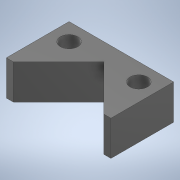
# Autodesk Inventor part: Subj_Cube
Saved by Autodesk Inventor 2021 (Build 250183000, 183)
## iProperties
Created: 2021-05-07
Part Number: Subj_Cube
Material: Genérico
Document SubType Name: Modeling
Designer: Marc
Density: 1 g/cm^3
Appearance: Valor por defecto
Author: Marc
## iProperties of the stored document _3DPrint.ipt
Created: 2021-05-07
Part Number: _3DPrint
Material: Genérico
Document SubType Name: Modeling
Designer: Marc
Density: 1 g/cm^3
Appearance: Valor por defecto
Author: Marc
Autodesk Inventor part; units mm, degrees
ref_plane "YZ Plane" through (0, 0, 0) normal (1, 0, 0) x (0, 1, 0)
ref_plane "XZ Plane" through (0, 0, 0) normal (0, 1, 0) x (-1, 0, 0)
ref_plane "XY Plane" through (0, 0, 0) normal (0, 0, 1) x (1, 0, 0)
sketch "Boceto1" plane through (0, 0, 0) normal (0, 1, 0) x (-1, 0, 0)
  line L0 (-15, -10) -> (15, -10)
  line L1 (13, 8) -> (0, -5)
  line L2 (-13, 8) -> (0, -5)
  line L3 (-15, 8) -> (-13, 8)
  line L4 (15, 8) -> (13, 8)
  line L5 (15, -10) -> (15, 8)
  line L6 (-15, -10) -> (-15, 8)
  line L7 (15, -10) -> (10, -10)
  line L8 (-15, -10) -> (-10, -10)
  circle A0 centre (-10, -5) radius 2.5
  circle A1 centre (10, -5) radius 2.5
  point P0 (0, 0)
  dimension "d5" = 5
  dimension "d8" = 5
  dimension "d9" = 5
  constraints: 18 end point, 2 centre point, 2 point on line, 1 horizontal, 1 parallel, 1 perpendicular, 1 vertical
  measures "d5" distance of L0.end L7.end
  measures "d8" diameter of A0
  measures "d9" diameter of A1
extrude "Extrusión1" add sketch "Boceto1" along normal blind 10
